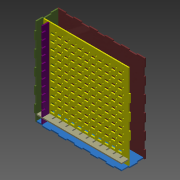
# Autodesk Inventor part: wordClock
Saved by Autodesk Inventor 2015 (Build 190159000, 159)
## iProperties
Created: 2015-02-10
Part Number: wordClock
Material: Generic
Document SubType Name: Modeling
Designer: Iain
Density: 1 g/cm^3
Appearance: Default
Author: Iain
Autodesk Inventor part; units mm, degrees
(part 1 of 2)
ref_plane "YZ Plane" through (0, 0, 0) normal (1, 0, 0) x (0, 1, 0)
ref_plane "XZ Plane" through (0, 0, 0) normal (0, 1, 0) x (-1, 0, 0)
ref_plane "XY Plane" through (0, 0, 0) normal (0, 0, 1) x (1, 0, 0)
sketch "Sketch1" plane through (0, 0, 0) normal (0, 0, 1) x (1, 0, 0)
  line L0 (-105, 105) -> (105, 105)
  line L1 (105, 105) -> (105, -105)
  line L2 (105, -105) -> (-105, -105)
  line L3 (-105, -105) -> (-105, 105)
  point P0 (0, 0)
  point P1 (0, 105)
  point P2 (-105, 0)
  dimension "FrontFaceBaseWidth" = 210
  dimension "FrontFaceBaseHeight" = 210
  constraints: 8 end point, 2 midpoint, 2 parallel, 1 horizontal, 1 horizontal alignment, 1 perpendicular, 1 vertical alignment
  measures "FrontFaceBaseWidth" distance of L0.start L0.end
  measures "FrontFaceBaseHeight" distance of L2.end L0.start
extrude "FrontFaceBase" add sketch "Sketch1" along normal mid plane 3
sketch "Sketch4" plane through (0, 0, 1.5) normal (0, 0, 1) x (1, 0, 0)
  line L0 (-108, 108) -> (-88, 108)
  line L1 (-88, 108) -> (-88, 105)
  line L2 (-88, 105) -> (-108, 105)
  line L3 (-108, 105) -> (-108, 108)
  point P0 (-105, 105)
  point P1 (0, 0)
  point P2 (-98, 105)
  dimension "d6" = 3
  dimension "FrontFaceTabWidth" = 20
  dimension "d8" = 3
  constraints: 8 end point, 2 parallel, 1 horizontal, 1 horizontal alignment, 1 midpoint, 1 perpendicular
  measures "d6" distance of point (-105, 105) L2.end
  measures "FrontFaceTabWidth" distance of L0.end L0.start
  measures "d8" distance of L1.end L0.end
extrude "Extrusion2" add sketch "Sketch4" against normal blind 3
pattern_linear "FrontTopTabs" count 6 spacing 39.2 along (1, 0, 0) of "Extrusion2"
sketch "Sketch5" plane through (0, 0, 1.5) normal (0, 0, 1) x (1, 0, 0)
  line L0 (-108, -108) -> (-105, -108)
  line L1 (-105, -108) -> (-105, -88)
  line L2 (-105, -88) -> (-108, -88)
  line L3 (-108, -88) -> (-108, -108)
  point P0 (-105, -105)
  point P1 (0, 0)
  point P2 (-105, -98)
  dimension "d14" = 3
  dimension "d15" = 3
  dimension "d16" = 20
  constraints: 8 end point, 2 parallel, 1 horizontal, 1 midpoint, 1 perpendicular, 1 vertical alignment
  measures "d14" distance of point (-105, -105) L0.end
  measures "d15" distance of L0.start L0.end
  measures "d16" distance of L2.end L0.start
extrude "Extrusion3" add sketch "Sketch5" against normal blind 3
pattern_linear "FontLeftTabs" count 6 spacing 39.2 along (0, 1, 0) of "Extrusion3"
mirror "FrontBottomTabs" about plane through (0, 0, 0) normal (0, 1, 0) of "Extrusion2", "FrontTopTabs"
mirror "FontRightTabs" about plane through (0, 0, 0) normal (1, 0, 0) of "Extrusion3", "FontLeftTabs"
sketch "Sketch6" plane through (-9.6, 105, -1.5) normal (0, 1, 0) x (1, 0, 0)
  line L0 (-98.4, -3) -> (117.6, -3)
  line L1 (117.6, -3) -> (117.6, 57)
  line L2 (117.6, 57) -> (-98.4, 57)
  line L3 (-98.4, 57) -> (-98.4, -3)
  line L4 (-59.2, -3) -> (-78.4, -3) projected
  line L5 (-98.4, -3) -> (-98.4, 0) projected
  point P0 (-98.4, -3)
  point P1 (117.6, 27)
  point P2 (9.6, -3)
  point P3 (-68.8, -3)
  point P4 (-98.4, 27)
  point P5 (-98.4, -1.5)
  dimension "d68" = 216
  dimension "d69" = 60
  constraints: 8 end point, 5 midpoint, 2 parallel, 1 horizontal, 1 horizontal alignment, 1 perpendicular, 1 vertical alignment
  measures "d68" distance of L0.start L0.end
  measures "d69" distance of L0.end L1.end
extrude "TopFaceBase" add sketch "Sketch6" along normal blind 3 separate body
sketch "Sketch7" plane through (-9.6, 108, -1.5) normal (0, 1, 0) x (1, 0, 0)
  line L0 (-98.4, -3) -> (117.6, -3) projected
  line L1 (-98.4, 57) -> (-98.4, -3) projected
  line L2 (-98.4, -3) -> (-78.4, -3)
  line L3 (-78.4, -3) -> (-78.4, 0)
  line L4 (-78.4, 0) -> (-98.4, 0)
  line L5 (-98.4, 0) -> (-98.4, -3)
  point P0 (9.6, -1.5)
  point P1 (-98.4, 27)
  point P2 (9.6, -3)
  dimension "d25" = 20
  dimension "TopFaceFrontSlotDepth" = 3
  constraints: 8 end point, 2 midpoint, 2 parallel, 1 horizontal, 1 horizontal alignment, 1 perpendicular, 1 vertical alignment
  measures "d25" distance of L3.end L4.end
  measures "TopFaceFrontSlotDepth" distance of L2.start L4.end
extrude "Extrusion5" cut sketch "Sketch7" against normal blind 3 bodies 2
sketch "Sketch8" plane through (-9.6, 108, -1.5) normal (0, 1, 0) x (1, 0, 0)
  line L0 (117.6, -3) -> (114.6, -3)
  line L1 (114.6, -3) -> (114.6, 17)
  line L2 (114.6, 17) -> (117.6, 17)
  line L3 (117.6, 17) -> (117.6, -3)
  point P0 (9.6, -1.5)
  dimension "TopSideSlotWidth" = 20
  dimension "d33" = 3
  constraints: 8 end point, 2 parallel, 1 horizontal, 1 perpendicular
  measures "TopSideSlotWidth" distance of L0.end L1.end
  measures "d33" distance of L0.start L0.end
extrude "Extrusion6" cut sketch "Sketch8" against normal blind 3 bodies 2
pattern_linear "TopFrontSlots" count 6 spacing 39.2 along (1, 0, 0) of "Extrusion5", "Extrusion2" bodies 2
pattern_linear "TopSideRightSlots" count 2 spacing 40 along (0, 0, -1) of "Extrusion6" bodies 2
ref_plane "Work Plane1" through (-48.8, 108, -28.5) normal (0, 0, 1) x (1, 0, 0)
mirror "TopBackSlots" about plane through (-48.8, 108, -28.5) normal (0, 0, 1) of "Extrusion5", "Extrusion2", "TopFrontSlots" bodies 2
ref_plane "Work Plane2" through (0, 105, -18.5) normal (1, 0, 0) x (0, 0, -1)
mirror "TopSideLeftSlots" about plane through (0, 105, -18.5) normal (1, 0, 0) of "Extrusion6", "TopSideRightSlots" bodies 2
sketch "Sketch12" plane through (108, 105, -18.5) normal (1, 0, 0) x (0, 0, -1)
  line L0 (0, 0) -> (20, 0) projected
  line L1 (-20, 0) -> (40, 0)
  line L2 (40, 0) -> (40, -210)
  line L3 (40, -210) -> (-20, -210)
  line L4 (-20, -210) -> (-20, 0)
  line L5 (-17, -95.4) -> (-17, -114.6) projected
  line L6 (-20, -114.6) -> (-20, -95.4) projected
  point P0 (-18.5, -105)
  point P1 (10, 0)
  point P2 (10, 0)
  point P3 (-20, -105)
  point P4 (-17, -105)
  point P5 (-20, -105)
  dimension "SideFaceBaseHeight" = 210
  dimension "SideFaceBaseDepth" = 60
  constraints: 8 end point, 5 midpoint, 2 coincident, 2 parallel, 1 horizontal, 1 perpendicular
  measures "SideFaceBaseHeight" distance of L3.end L1.start
  measures "SideFaceBaseDepth" distance of L1.start L1.end
extrude "RightFaceBase" add sketch "Sketch12" against normal blind 3 separate body
sketch "Sketch13" plane through (108, 105, -18.5) normal (1, 0, 0) x (0, 0, -1)
  line L0 (-20, 0) -> (40, 0) projected
  line L1 (-20, 3) -> (0, 3)
  line L2 (0, 3) -> (0, 0)
  line L3 (0, 0) -> (-20, 0)
  line L4 (-20, 0) -> (-20, 3)
  line L5 (-20, -114.6) -> (-20, -95.4) projected
  point P0 (-18.5, -105)
  point P1 (-10, 0)
  point P2 (10, 0)
  point P3 (-20, 1.5)
  point P4 (-20, -105)
  dimension "SideFaceTabWidth" = 20
  dimension "SideTopTabDepth" = 3
  constraints: 8 end point, 4 midpoint, 2 parallel, 1 horizontal, 1 horizontal alignment, 1 perpendicular, 1 vertical alignment
  measures "SideFaceTabWidth" distance of L1.start L1.end
  measures "SideTopTabDepth" distance of L3.end L1.start
extrude "Extrusion9" add sketch "Sketch13" against normal blind 3 bodies 3
pattern_linear "SideTopTabs" count 2 spacing 40 along (0, 0, -1) of "Extrusion9" bodies 3
mirror "SideBottomTabs" about plane through (0, 0, 0) normal (0, 1, 0) of "Extrusion9", "SideTopTabs" bodies 3
sketch "Sketch14" plane through (108, 105, -18.5) normal (1, 0, 0) x (0, 0, -1)
  line L0 (-20, 3) -> (-20, -213) projected
  line L1 (-20, 3) -> (0, 3) projected
  line L2 (-20, 3) -> (-17, 3)
  line L3 (-17, 3) -> (-17, -17)
  line L4 (-17, -17) -> (-20, -17)
  line L5 (-20, -17) -> (-20, 3)
  point P0 (-18.5, -105)
  point P1 (-18.5, 3)
  point P2 (-10, 3)
  point P3 (-20, -7)
  point P4 (-20, -105)
  dimension "d61" = 3
  dimension "d62" = 20
  constraints: 8 end point, 4 midpoint, 2 parallel, 1 horizontal, 1 horizontal alignment, 1 perpendicular, 1 vertical alignment
  measures "d61" distance of L2.start L2.end
  measures "d62" distance of L4.end L2.start
extrude "Extrusion10" cut sketch "Sketch14" against normal blind 3 bodies 3
pattern_linear "SideFrontSlots" count 6 spacing 39.2 along (0, -1, 0) of "Extrusion10" bodies 3
ref_plane "Work Plane4" through (105, 29.6, -28.5) normal (0, 0, 1) x (1, 0, 0)
mirror "SideBackSlots" about plane through (105, 29.6, -28.5) normal (0, 0, 1) of "Extrusion10", "SideFrontSlots" bodies 3
mirror "Back" about plane through (105, 29.6, -28.5) normal (0, 0, 1) bodies 1 separate body
mirror "Left" about plane through (0, 105, -18.5) normal (1, 0, 0) bodies 3 separate body
mirror "Bottom" about plane through (0, 0, 0) normal (0, 1, 0) bodies 2 separate body
ref_plane "MiddleFacePlane" through (0, 0, -18.5) normal (0, 0, 1) x (1, 0, 0)
sketch "Sketch17" plane through (0, 0, -18.5) normal (0, 0, 1) x (1, 0, 0)
  line L0 (-105, 105) -> (105, 105)
  line L1 (105, 105) -> (105, -105)
  line L2 (105, -105) -> (-105, -105)
  line L3 (-105, -105) -> (-105, 105)
  point P0 (0, 0)
  point P1 (0, 105)
  point P2 (105, 0)
  dimension "d76" = 210
  dimension "d77" = 210
  constraints: 8 end point, 2 midpoint, 2 parallel, 1 horizontal, 1 horizontal alignment, 1 perpendicular, 1 vertical alignment
  measures "d76" distance of L0.end L1.end
  measures "d77" distance of L0.start L0.end
extrude "Extrusion13" add sketch "Sketch17" against normal blind 3 separate body
sketch "Sketch18" plane through (0, 0, -18.5) normal (0, 0, 1) x (1, 0, 0)
  line L0 (-105, -105) -> (-105, 105) projected
  line L1 (-105, -10) -> (-108, -10)
  line L2 (-108, -10) -> (-108, 10)
  line L3 (-108, 10) -> (-105, 10)
  line L4 (-105, 10) -> (-105, -10)
  point P0 (0, 0)
  point P1 (-105, 0)
  point P2 (-105, 0)
  point P3 (-108, 0)
  dimension "d80" = 3
  dimension "MiddleTabWidth" = 20
  constraints: 8 end point, 3 midpoint, 2 parallel, 1 coincident, 1 horizontal, 1 horizontal alignment, 1 perpendicular
  measures "d80" distance of L2.end L3.end
  measures "MiddleTabWidth" distance of L1.end L2.end
extrude "Extrusion14" add sketch "Sketch18" against normal blind 3 bodies 7
pattern_linear "LeftMiddleTabs" count 3 spacing 40 along (0, 1, 0) of "Extrusion14" first direction both ways yes bodies 7
mirror "RightMiddleTabs" about plane through (0, 0, 0) normal (1, 0, 0) of "Extrusion14", "LeftMiddleTabs" bodies 7
sketch "Sketch19" plane through (0, 0, -18.5) normal (0, 0, 1) x (1, 0, 0)
  line L0 (105, -105) -> (-105, -105) projected
  line L1 (-10, -105) -> (10, -105)
  line L2 (10, -105) -> (10, -108)
  line L3 (10, -108) -> (-10, -108)
  line L4 (-10, -108) -> (-10, -105)
  point P0 (0, 0)
  point P1 (0, -105)
  point P2 (0, -105)
  dimension "d87" = 3
  dimension "MiddleBottomTabWidth" = 20
  constraints: 8 end point, 2 midpoint, 2 parallel, 1 coincident, 1 horizontal, 1 perpendicular, 1 vertical alignment
  measures "d87" distance of L1.end L2.end
  measures "MiddleBottomTabWidth" distance of L1.start L1.end
extrude "Extrusion15" add sketch "Sketch19" against normal blind 3 bodies 7
pattern_linear "Rectangular Pattern9" count 3 spacing 40 along (-1, 0, 0) of "Extrusion15" first direction both ways yes bodies 7
sketch "Sketch21" plane through (0, 0, -18.5) normal (0, 0, 1) x (1, 0, 0)
  line L0 (10, -108) -> (-10, -108) projected
  line L1 (-10, -105) -> (10, -105)
  line L2 (10, -105) -> (10, -108)
  line L3 (10, -108) -> (-10, -108)
  line L4 (-10, -108) -> (-10, -105)
  point P0 (0, 0)
  point P1 (0, -105)
  point P2 (0, -108)
  point P3 (0, -108)
  dimension "d94" = 3
  dimension "d95" = 20
  constraints: 8 end point, 3 midpoint, 2 parallel, 1 coincident, 1 horizontal, 1 perpendicular, 1 vertical alignment
  measures "d94" distance of L1.end L2.end
  measures "d95" distance of L1.start L1.end
extrude "Extrusion16" cut sketch "Sketch21" against normal blind 3 bodies 6
pattern_linear "BottomMiddleSlots" count 3 spacing 40 along (-1, 0, 0) of "Extrusion16" first direction both ways yes bodies 6
sketch "Sketch22" plane through (0, 0, -18.5) normal (0, 0, 1) x (1, 0, 0)
  line L0 (-108, -10) -> (-108, 10) projected
  line L1 (-108, 10) -> (-105, 10)
  line L2 (-105, 10) -> (-105, -10)
  line L3 (-105, -10) -> (-108, -10)
  line L4 (-108, -10) -> (-108, 10)
  point P0 (0, 0)
  point P1 (-105, 0)
  point P2 (-108, 0)
  point P3 (-108, 0)
  dimension "d101" = 3
  dimension "d102" = 20
  constraints: 8 end point, 3 midpoint, 2 parallel, 1 coincident, 1 horizontal, 1 horizontal alignment, 1 perpendicular
  measures "d101" distance of L1.end L1.start
  measures "d102" distance of L3.end L1.start
extrude "Extrusion17" cut sketch "Sketch22" against normal blind 3 bodies 5
pattern_linear "LeftMiddleSlots" count 3 spacing 40 along (0, 1, 0) of "Extrusion14", "Extrusion17" first direction both ways yes bodies 5
mirror "RightMiddleSlots" about plane through (0, 0, 0) normal (1, 0, 0) of "LeftMiddleSlots", "Extrusion14", "Extrusion17" bodies 3
sketch "gridConstruct" plane through (0, 0, 1.5) normal (0, 0, 1) x (1, 0, 0)
  line L0 (88, 108) -> (108, 108) projected
  line L1 (88, 105) -> (88, 108) projected
  line L2 (88, 105) -> (68.8, 105) projected
  line L3 (68.8, 108) -> (68.8, 105) projected
  line L4 (48.8, 108) -> (68.8, 108) projected
  line L5 (48.8, 105) -> (48.8, 108) projected
  line L6 (48.8, 105) -> (29.6, 105) projected
  line L7 (29.6, 108) -> (29.6, 105) projected
  line L8 (9.6, 108) -> (29.6, 108) projected
  line L9 (9.6, 105) -> (9.6, 108) projected
  line L10 (9.6, 105) -> (-9.6, 105) projected
  line L11 (-9.6, 108) -> (-9.6, 105) projected
  line L12 (-29.6, 108) -> (-9.6, 108) projected
  line L13 (-29.6, 105) -> (-29.6, 108) projected
  line L14 (-29.6, 105) -> (-48.8, 105) projected
  line L15 (-48.8, 108) -> (-48.8, 105) projected
  line L16 (-68.8, 108) -> (-48.8, 108) projected
  line L17 (-68.8, 105) -> (-68.8, 108) projected
  line L18 (-68.8, 105) -> (-88, 105) projected
  line L19 (-88, 108) -> (-88, 105) projected
  line L20 (-108, 108) -> (-88, 108) projected
  line L21 (-108, 108) -> (-108, 88) projected
  line L22 (-108, 88) -> (-105, 88) projected
  line L23 (-105, 88) -> (-105, 68.8) projected
  line L24 (-105, 68.8) -> (-108, 68.8) projected
  line L25 (-108, 68.8) -> (-108, 48.8) projected
  line L26 (-108, 48.8) -> (-105, 48.8) projected
  line L27 (-105, 48.8) -> (-105, 29.6) projected
  line L28 (-105, 29.6) -> (-108, 29.6) projected
  line L29 (-108, 29.6) -> (-108, 9.6) projected
  line L30 (-108, 9.6) -> (-105, 9.6) projected
  line L31 (-105, 9.6) -> (-105, -9.6) projected
  line L32 (-105, -9.6) -> (-108, -9.6) projected
  line L33 (-108, -9.6) -> (-108, -29.6) projected
  line L34 (-108, -29.6) -> (-105, -29.6) projected
  line L35 (-105, -29.6) -> (-105, -48.8) projected
  line L36 (-105, -48.8) -> (-108, -48.8) projected
  line L37 (-108, -48.8) -> (-108, -68.8) projected
  line L38 (-108, -68.8) -> (-105, -68.8) projected
  line L39 (-105, -68.8) -> (-105, -88) projected
  line L40 (-105, -88) -> (-108, -88) projected
  line L41 (-108, -88) -> (-108, -108) projected
  line L42 (-108, -108) -> (-88, -108) projected
  line L43 (-88, -108) -> (-88, -105) projected
  line L44 (-88, -105) -> (-68.8, -105) projected
  line L45 (-68.8, -105) -> (-68.8, -108) projected
  line L46 (-68.8, -108) -> (-48.8, -108) projected
  line L47 (-48.8, -108) -> (-48.8, -105) projected
  line L48 (-48.8, -105) -> (-29.6, -105) projected
  line L49 (-29.6, -105) -> (-29.6, -108) projected
  line L50 (-29.6, -108) -> (-9.6, -108) projected
  line L51 (-9.6, -108) -> (-9.6, -105) projected
  line L52 (-9.6, -105) -> (9.6, -105) projected
  line L53 (9.6, -105) -> (9.6, -108) projected
  line L54 (9.6, -108) -> (29.6, -108) projected
  line L55 (29.6, -108) -> (29.6, -105) projected
  line L56 (29.6, -105) -> (48.8, -105) projected
  line L57 (48.8, -105) -> (48.8, -108) projected
  line L58 (48.8, -108) -> (68.8, -108) projected
  line L59 (68.8, -108) -> (68.8, -105) projected
  line L60 (68.8, -105) -> (88, -105) projected
  line L61 (88, -105) -> (88, -108) projected
  line L62 (88, -108) -> (108, -108) projected
  line L63 (108, -108) -> (108, -88) projected
  line L64 (105, -88) -> (108, -88) projected
  line L65 (105, -88) -> (105, -68.8) projected
  line L66 (108, -68.8) -> (105, -68.8) projected
  line L67 (108, -48.8) -> (108, -68.8) projected
  line L68 (105, -48.8) -> (108, -48.8) projected
  line L69 (105, -48.8) -> (105, -29.6) projected
  line L70 (108, -29.6) -> (105, -29.6) projected
  line L71 (108, -9.6) -> (108, -29.6) projected
  line L72 (105, -9.6) -> (108, -9.6) projected
  line L73 (105, -9.6) -> (105, 9.6) projected
  line L74 (108, 9.6) -> (105, 9.6) projected
  line L75 (108, 29.6) -> (108, 9.6) projected
  line L76 (105, 29.6) -> (108, 29.6) projected
  line L77 (105, 29.6) -> (105, 48.8) projected
  line L78 (108, 48.8) -> (105, 48.8) projected
  line L79 (108, 68.8) -> (108, 48.8) projected
  line L80 (105, 68.8) -> (108, 68.8) projected
  line L81 (105, 68.8) -> (105, 88) projected
  line L82 (108, 88) -> (105, 88) projected
  line L83 (108, 108) -> (108, 88) projected
  line L84 (-91.6667, -75) -> (-75, -75) construction
  line L85 (-75, -75) -> (-75, -91.6667) construction
  line L86 (-75, -91.6667) -> (-91.6667, -91.6667) construction
  line L87 (-91.6667, -91.6667) -> (-91.6667, -75) construction
  line L88 (-75, -75) -> (-58.3333, -75) construction
  line L89 (-58.3333, -75) -> (-58.3333, -91.6667) construction
  line L90 (-58.3333, -91.6667) -> (-75, -91.6667) construction
  line L91 (-75, -91.6667) -> (-75, -75) construction
  line L92 (-58.3333, -75) -> (-41.6667, -75) construction
  line L93 (-41.6667, -75) -> (-41.6667, -91.6667) construction
  line L94 (-41.6667, -91.6667) -> (-58.3333, -91.6667) construction
  line L95 (-58.3333, -91.6667) -> (-58.3333, -75) construction
  line L96 (-41.6667, -75) -> (-25, -75) construction
  line L97 (-25, -75) -> (-25, -91.6667) construction
  line L98 (-25, -91.6667) -> (-41.6667, -91.6667) construction
  line L99 (-41.6667, -91.6667) -> (-41.6667, -75) construction
  line L100 (-25, -75) -> (-8.3333, -75) construction
  line L101 (-8.3333, -75) -> (-8.3333, -91.6667) construction
  line L102 (-8.3333, -91.6667) -> (-25, -91.6667) construction
  line L103 (-25, -91.6667) -> (-25, -75) construction
  line L104 (-8.3333, -75) -> (8.3333, -75) construction
  line L105 (8.3333, -75) -> (8.3333, -91.6667) construction
  line L106 (8.3333, -91.6667) -> (-8.3333, -91.6667) construction
  line L107 (-8.3333, -91.6667) -> (-8.3333, -75) construction
  line L108 (-91.6667, -58.3333) -> (-75, -58.3333) construction
  line L109 (-75, -58.3333) -> (-75, -75) construction
  line L110 (-75, -75) -> (-91.6667, -75) construction
  line L111 (-91.6667, -75) -> (-91.6667, -58.3333) construction
  line L112 (-75, -58.3333) -> (-58.3333, -58.3333) construction
  line L113 (-58.3333, -58.3333) -> (-58.3333, -75) construction
  line L114 (-58.3333, -75) -> (-75, -75) construction
  line L115 (-75, -75) -> (-75, -58.3333) construction
  line L116 (-58.3333, -58.3333) -> (-41.6667, -58.3333) construction
  line L117 (-41.6667, -58.3333) -> (-41.6667, -75) construction
  line L118 (-41.6667, -75) -> (-58.3333, -75) construction
  line L119 (-58.3333, -75) -> (-58.3333, -58.3333) construction
  line L120 (-41.6667, -58.3333) -> (-25, -58.3333) construction
  line L121 (-25, -58.3333) -> (-25, -75) construction
  line L122 (-25, -75) -> (-41.6667, -75) construction
  line L123 (-41.6667, -75) -> (-41.6667, -58.3333) construction
  line L124 (-25, -58.3333) -> (-8.3333, -58.3333) construction
  line L125 (-8.3333, -58.3333) -> (-8.3333, -75) construction
  line L126 (-8.3333, -75) -> (-25, -75) construction
  line L127 (-25, -75) -> (-25, -58.3333) construction
  line L128 (-8.3333, -58.3333) -> (8.3333, -58.3333) construction
  line L129 (8.3333, -58.3333) -> (8.3333, -75) construction
  line L130 (8.3333, -75) -> (-8.3333, -75) construction
  line L131 (-8.3333, -75) -> (-8.3333, -58.3333) construction
  line L132 (-91.6667, -41.6667) -> (-75, -41.6667) construction
  line L133 (-75, -41.6667) -> (-75, -58.3333) construction
  line L134 (-75, -58.3333) -> (-91.6667, -58.3333) construction
  line L135 (-91.6667, -58.3333) -> (-91.6667, -41.6667) construction
  line L136 (-75, -41.6667) -> (-58.3333, -41.6667) construction
  line L137 (-58.3333, -41.6667) -> (-58.3333, -58.3333) construction
  line L138 (-58.3333, -58.3333) -> (-75, -58.3333) construction
  line L139 (-75, -58.3333) -> (-75, -41.6667) construction
  line L140 (-58.3333, -41.6667) -> (-41.6667, -41.6667) construction
  line L141 (-41.6667, -41.6667) -> (-41.6667, -58.3333) construction
  line L142 (-41.6667, -58.3333) -> (-58.3333, -58.3333) construction
  line L143 (-58.3333, -58.3333) -> (-58.3333, -41.6667) construction
  line L144 (-41.6667, -41.6667) -> (-25, -41.6667) construction
  line L145 (-25, -41.6667) -> (-25, -58.3333) construction
  line L146 (-25, -58.3333) -> (-41.6667, -58.3333) construction
  line L147 (-41.6667, -58.3333) -> (-41.6667, -41.6667) construction
  line L148 (-25, -41.6667) -> (-8.3333, -41.6667) construction
  line L149 (-8.3333, -41.6667) -> (-8.3333, -58.3333) construction
  line L150 (-8.3333, -58.3333) -> (-25, -58.3333) construction
  line L151 (-25, -58.3333) -> (-25, -41.6667) construction
  line L152 (-8.3333, -41.6667) -> (8.3333, -41.6667) construction
  line L153 (8.3333, -41.6667) -> (8.3333, -58.3333) construction
  line L154 (8.3333, -58.3333) -> (-8.3333, -58.3333) construction
  line L155 (-8.3333, -58.3333) -> (-8.3333, -41.6667) construction
  line L156 (-91.6667, -25) -> (-75, -25) construction
  line L157 (-75, -25) -> (-75, -41.6667) construction
  line L158 (-75, -41.6667) -> (-91.6667, -41.6667) construction
  line L159 (-91.6667, -41.6667) -> (-91.6667, -25) construction
  line L160 (-75, -25) -> (-58.3333, -25) construction
  line L161 (-58.3333, -25) -> (-58.3333, -41.6667) construction
  line L162 (-58.3333, -41.6667) -> (-75, -41.6667) construction
  line L163 (-75, -41.6667) -> (-75, -25) construction
  line L164 (-58.3333, -25) -> (-41.6667, -25) construction
  line L165 (-41.6667, -25) -> (-41.6667, -41.6667) construction
  line L166 (-41.6667, -41.6667) -> (-58.3333, -41.6667) construction
  line L167 (-58.3333, -41.6667) -> (-58.3333, -25) construction
  line L168 (-41.6667, -25) -> (-25, -25) construction
  line L169 (-25, -25) -> (-25, -41.6667) construction
  line L170 (-25, -41.6667) -> (-41.6667, -41.6667) construction
  line L171 (-41.6667, -41.6667) -> (-41.6667, -25) construction
  line L172 (-25, -25) -> (-8.3333, -25) construction
  line L173 (-8.3333, -25) -> (-8.3333, -41.6667) construction
  line L174 (-8.3333, -41.6667) -> (-25, -41.6667) construction
  line L175 (-25, -41.6667) -> (-25, -25) construction
  line L176 (-8.3333, -25) -> (8.3333, -25) construction
  line L177 (8.3333, -25) -> (8.3333, -41.6667) construction
  line L178 (8.3333, -41.6667) -> (-8.3333, -41.6667) construction
  line L179 (-8.3333, -41.6667) -> (-8.3333, -25) construction
  line L180 (-91.6667, -8.3333) -> (-75, -8.3333) construction
  line L181 (-75, -8.3333) -> (-75, -25) construction
  line L182 (-75, -25) -> (-91.6667, -25) construction
  line L183 (-91.6667, -25) -> (-91.6667, -8.3333) construction
  line L184 (-75, -8.3333) -> (-58.3333, -8.3333) construction
  line L185 (-58.3333, -8.3333) -> (-58.3333, -25) construction
  line L186 (-58.3333, -25) -> (-75, -25) construction
  line L187 (-75, -25) -> (-75, -8.3333) construction
  line L188 (-58.3333, -8.3333) -> (-41.6667, -8.3333) construction
  line L189 (-41.6667, -8.3333) -> (-41.6667, -25) construction
  line L190 (-41.6667, -25) -> (-58.3333, -25) construction
  line L191 (-58.3333, -25) -> (-58.3333, -8.3333) construction
  line L192 (-41.6667, -8.3333) -> (-25, -8.3333) construction
  line L193 (-25, -8.3333) -> (-25, -25) construction
  line L194 (-25, -25) -> (-41.6667, -25) construction
  line L195 (-41.6667, -25) -> (-41.6667, -8.3333) construction
  line L196 (-25, -8.3333) -> (-8.3333, -8.3333) construction
  line L197 (-8.3333, -8.3333) -> (-8.3333, -25) construction
  line L198 (-8.3333, -25) -> (-25, -25) construction
  line L199 (-25, -25) -> (-25, -8.3333) construction
  line L200 (-8.3333, -8.3333) -> (8.3333, -8.3333) construction
  line L201 (8.3333, -8.3333) -> (8.3333, -25) construction
  line L202 (8.3333, -25) -> (-8.3333, -25) construction
  line L203 (-8.3333, -25) -> (-8.3333, -8.3333) construction
  line L204 (-91.6667, 8.3333) -> (-75, 8.3333) construction
  line L205 (-75, 8.3333) -> (-75, -8.3333) construction
  line L206 (-75, -8.3333) -> (-91.6667, -8.3333) construction
  line L207 (-91.6667, -8.3333) -> (-91.6667, 8.3333) construction
  line L208 (-75, 8.3333) -> (-58.3333, 8.3333) construction
  line L209 (-58.3333, 8.3333) -> (-58.3333, -8.3333) construction
  line L210 (-58.3333, -8.3333) -> (-75, -8.3333) construction
  line L211 (-75, -8.3333) -> (-75, 8.3333) construction
  line L212 (-58.3333, 8.3333) -> (-41.6667, 8.3333) construction
  line L213 (-41.6667, 8.3333) -> (-41.6667, -8.3333) construction
  line L214 (-41.6667, -8.3333) -> (-58.3333, -8.3333) construction
  line L215 (-58.3333, -8.3333) -> (-58.3333, 8.3333) construction
  line L216 (-41.6667, 8.3333) -> (-25, 8.3333) construction
  line L217 (-25, 8.3333) -> (-25, -8.3333) construction
  line L218 (-25, -8.3333) -> (-41.6667, -8.3333) construction
  line L219 (-41.6667, -8.3333) -> (-41.6667, 8.3333) construction
  line L220 (-25, 8.3333) -> (-8.3333, 8.3333) construction
  line L221 (-8.3333, 8.3333) -> (-8.3333, -8.3333) construction
  line L222 (-8.3333, -8.3333) -> (-25, -8.3333) construction
  line L223 (-25, -8.3333) -> (-25, 8.3333) construction
  line L224 (-8.3333, 8.3333) -> (8.3333, 8.3333) construction
  line L225 (8.3333, 8.3333) -> (8.3333, -8.3333) construction
  line L226 (8.3333, -8.3333) -> (-8.3333, -8.3333) construction
  line L227 (-8.3333, -8.3333) -> (-8.3333, 8.3333) construction
  line L228 (-91.6667, 25) -> (-75, 25) construction
  line L229 (-75, 25) -> (-75, 8.3333) construction
  line L230 (-75, 8.3333) -> (-91.6667, 8.3333) construction
  line L231 (-91.6667, 8.3333) -> (-91.6667, 25) construction
  line L232 (-75, 25) -> (-58.3333, 25) construction
  line L233 (-58.3333, 25) -> (-58.3333, 8.3333) construction
  line L234 (-58.3333, 8.3333) -> (-75, 8.3333) construction
  line L235 (-75, 8.3333) -> (-75, 25) construction
  line L236 (-58.3333, 25) -> (-41.6667, 25) construction
  line L237 (-41.6667, 25) -> (-41.6667, 8.3333) construction
  line L238 (-41.6667, 8.3333) -> (-58.3333, 8.3333) construction
  line L239 (-58.3333, 8.3333) -> (-58.3333, 25) construction
  line L240 (-41.6667, 25) -> (-25, 25) construction
  line L241 (-25, 25) -> (-25, 8.3333) construction
  line L242 (-25, 8.3333) -> (-41.6667, 8.3333) construction
  line L243 (-41.6667, 8.3333) -> (-41.6667, 25) construction
  line L244 (-25, 25) -> (-8.3333, 25) construction
  line L245 (-8.3333, 25) -> (-8.3333, 8.3333) construction
  line L246 (-8.3333, 8.3333) -> (-25, 8.3333) construction
  line L247 (-25, 8.3333) -> (-25, 25) construction
  line L248 (-8.3333, 25) -> (8.3333, 25) construction
  line L249 (8.3333, 25) -> (8.3333, 8.3333) construction
  line L250 (8.3333, 8.3333) -> (-8.3333, 8.3333) construction
  line L251 (-8.3333, 8.3333) -> (-8.3333, 25) construction
  line L252 (-91.6667, 41.6667) -> (-75, 41.6667) construction
  line L253 (-75, 41.6667) -> (-75, 25) construction
  line L254 (-75, 25) -> (-91.6667, 25) construction
  line L255 (-91.6667, 25) -> (-91.6667, 41.6667) construction
  line L256 (-75, 41.6667) -> (-58.3333, 41.6667) construction
  line L257 (-58.3333, 41.6667) -> (-58.3333, 25) construction
  line L258 (-58.3333, 25) -> (-75, 25) construction
  line L259 (-75, 25) -> (-75, 41.6667) construction
  line L260 (-58.3333, 41.6667) -> (-41.6667, 41.6667) construction
  line L261 (-41.6667, 41.6667) -> (-41.6667, 25) construction
  line L262 (-41.6667, 25) -> (-58.3333, 25) construction
  line L263 (-58.3333, 25) -> (-58.3333, 41.6667) construction
  line L264 (-41.6667, 41.6667) -> (-25, 41.6667) construction
  line L265 (-25, 41.6667) -> (-25, 25) construction
  line L266 (-25, 25) -> (-41.6667, 25) construction
  line L267 (-41.6667, 25) -> (-41.6667, 41.6667) construction
  line L268 (-25, 41.6667) -> (-8.3333, 41.6667) construction
  line L269 (-8.3333, 41.6667) -> (-8.3333, 25) construction
  line L270 (-8.3333, 25) -> (-25, 25) construction
  line L271 (-25, 25) -> (-25, 41.6667) construction
  line L272 (-8.3333, 41.6667) -> (8.3333, 41.6667) construction
  line L273 (8.3333, 41.6667) -> (8.3333, 25) construction
  line L274 (8.3333, 25) -> (-8.3333, 25) construction
  line L275 (-8.3333, 25) -> (-8.3333, 41.6667) construction
  line L276 (-91.6667, 58.3333) -> (-75, 58.3333) construction
  line L277 (-75, 58.3333) -> (-75, 41.6667) construction
  line L278 (-75, 41.6667) -> (-91.6667, 41.6667) construction
  line L279 (-91.6667, 41.6667) -> (-91.6667, 58.3333) construction
  line L280 (-75, 58.3333) -> (-58.3333, 58.3333) construction
  line L281 (-58.3333, 58.3333) -> (-58.3333, 41.6667) construction
  line L282 (-58.3333, 41.6667) -> (-75, 41.6667) construction
  line L283 (-75, 41.6667) -> (-75, 58.3333) construction
  line L284 (-58.3333, 58.3333) -> (-41.6667, 58.3333) construction
  line L285 (-41.6667, 58.3333) -> (-41.6667, 41.6667) construction
  line L286 (-41.6667, 41.6667) -> (-58.3333, 41.6667) construction
  line L287 (-58.3333, 41.6667) -> (-58.3333, 58.3333) construction
  line L288 (-41.6667, 58.3333) -> (-25, 58.3333) construction
  line L289 (-25, 58.3333) -> (-25, 41.6667) construction
  line L290 (-25, 41.6667) -> (-41.6667, 41.6667) construction
  line L291 (-41.6667, 41.6667) -> (-41.6667, 58.3333) construction
  line L292 (-25, 58.3333) -> (-8.3333, 58.3333) construction
  line L293 (-8.3333, 58.3333) -> (-8.3333, 41.6667) construction
  line L294 (-8.3333, 41.6667) -> (-25, 41.6667) construction
  line L295 (-25, 41.6667) -> (-25, 58.3333) construction
  line L296 (-8.3333, 58.3333) -> (8.3333, 58.3333) construction
  line L297 (8.3333, 58.3333) -> (8.3333, 41.6667) construction
  line L298 (8.3333, 41.6667) -> (-8.3333, 41.6667) construction
  line L299 (-8.3333, 41.6667) -> (-8.3333, 58.3333) construction
  line L300 (8.3333, -75) -> (25, -75) construction
  line L301 (25, -75) -> (25, -91.6667) construction
  line L302 (25, -91.6667) -> (8.3333, -91.6667) construction
  line L303 (8.3333, -91.6667) -> (8.3333, -75) construction
  line L304 (8.3333, -58.3333) -> (25, -58.3333) construction
  line L305 (25, -58.3333) -> (25, -75) construction
  line L306 (25, -75) -> (8.3333, -75) construction
  line L307 (8.3333, -75) -> (8.3333, -58.3333) construction
  line L308 (8.3333, -41.6667) -> (25, -41.6667) construction
  line L309 (25, -41.6667) -> (25, -58.3333) construction
  line L310 (25, -58.3333) -> (8.3333, -58.3333) construction
  line L311 (8.3333, -58.3333) -> (8.3333, -41.6667) construction
  line L312 (8.3333, -25) -> (25, -25) construction
  line L313 (25, -25) -> (25, -41.6667) construction
  line L314 (25, -41.6667) -> (8.3333, -41.6667) construction
  line L315 (8.3333, -41.6667) -> (8.3333, -25) construction
  line L316 (8.3333, -8.3333) -> (25, -8.3333) construction
  line L317 (25, -8.3333) -> (25, -25) construction
  line L318 (25, -25) -> (8.3333, -25) construction
  line L319 (8.3333, -25) -> (8.3333, -8.3333) construction
  line L320 (8.3333, 8.3333) -> (25, 8.3333) construction
  line L321 (25, 8.3333) -> (25, -8.3333) construction
  line L322 (25, -8.3333) -> (8.3333, -8.3333) construction
  line L323 (8.3333, -8.3333) -> (8.3333, 8.3333) construction
  line L324 (8.3333, 25) -> (25, 25) construction
  line L325 (25, 25) -> (25, 8.3333) construction
  line L326 (25, 8.3333) -> (8.3333, 8.3333) construction
  line L327 (8.3333, 8.3333) -> (8.3333, 25) construction
  line L328 (8.3333, 41.6667) -> (25, 41.6667) construction
  line L329 (25, 41.6667) -> (25, 25) construction
  line L330 (25, 25) -> (8.3333, 25) construction
  line L331 (8.3333, 25) -> (8.3333, 41.6667) construction
  line L332 (8.3333, 58.3333) -> (25, 58.3333) construction
  line L333 (25, 58.3333) -> (25, 41.6667) construction
  line L334 (25, 41.6667) -> (8.3333, 41.6667) construction
  line L335 (8.3333, 41.6667) -> (8.3333, 58.3333) construction
  line L336 (25, -75) -> (41.6667, -75) construction
  line L337 (41.6667, -75) -> (41.6667, -91.6667) construction
  line L338 (41.6667, -91.6667) -> (25, -91.6667) construction
  line L339 (25, -91.6667) -> (25, -75) construction
  line L340 (25, -58.3333) -> (41.6667, -58.3333) construction
  line L341 (41.6667, -58.3333) -> (41.6667, -75) construction
  line L342 (41.6667, -75) -> (25, -75) construction
  line L343 (25, -75) -> (25, -58.3333) construction
  line L344 (25, -41.6667) -> (41.6667, -41.6667) construction
  line L345 (41.6667, -41.6667) -> (41.6667, -58.3333) construction
  line L346 (41.6667, -58.3333) -> (25, -58.3333) construction
  line L347 (25, -58.3333) -> (25, -41.6667) construction
  line L348 (25, -25) -> (41.6667, -25) construction
  line L349 (41.6667, -25) -> (41.6667, -41.6667) construction
  line L350 (41.6667, -41.6667) -> (25, -41.6667) construction
  line L351 (25, -41.6667) -> (25, -25) construction
  line L352 (25, -8.3333) -> (41.6667, -8.3333) construction
  line L353 (41.6667, -8.3333) -> (41.6667, -25) construction
  line L354 (41.6667, -25) -> (25, -25) construction
  line L355 (25, -25) -> (25, -8.3333) construction
  line L356 (25, 8.3333) -> (41.6667, 8.3333) construction
  line L357 (41.6667, 8.3333) -> (41.6667, -8.3333) construction
  line L358 (41.6667, -8.3333) -> (25, -8.3333) construction
  line L359 (25, -8.3333) -> (25, 8.3333) construction
  line L360 (25, 25) -> (41.6667, 25) construction
  line L361 (41.6667, 25) -> (41.6667, 8.3333) construction
  line L362 (41.6667, 8.3333) -> (25, 8.3333) construction
  line L363 (25, 8.3333) -> (25, 25) construction
  line L364 (25, 41.6667) -> (41.6667, 41.6667) construction
  line L365 (41.6667, 41.6667) -> (41.6667, 25) construction
  line L366 (41.6667, 25) -> (25, 25) construction
  line L367 (25, 25) -> (25, 41.6667) construction
  line L368 (25, 58.3333) -> (41.6667, 58.3333) construction
  line L369 (41.6667, 58.3333) -> (41.6667, 41.6667) construction
  line L370 (41.6667, 41.6667) -> (25, 41.6667) construction
  line L371 (25, 41.6667) -> (25, 58.3333) construction
  line L372 (41.6667, -75) -> (58.3333, -75) construction
  line L373 (58.3333, -75) -> (58.3333, -91.6667) construction
  line L374 (58.3333, -91.6667) -> (41.6667, -91.6667) construction
  line L375 (41.6667, -91.6667) -> (41.6667, -75) construction
  line L376 (41.6667, -58.3333) -> (58.3333, -58.3333) construction
  line L377 (58.3333, -58.3333) -> (58.3333, -75) construction
  line L378 (58.3333, -75) -> (41.6667, -75) construction
  line L379 (41.6667, -75) -> (41.6667, -58.3333) construction
  line L380 (41.6667, -41.6667) -> (58.3333, -41.6667) construction
  line L381 (58.3333, -41.6667) -> (58.3333, -58.3333) construction
  line L382 (58.3333, -58.3333) -> (41.6667, -58.3333) construction
  line L383 (41.6667, -58.3333) -> (41.6667, -41.6667) construction
  line L384 (41.6667, -25) -> (58.3333, -25) construction
  line L385 (58.3333, -25) -> (58.3333, -41.6667) construction
  line L386 (58.3333, -41.6667) -> (41.6667, -41.6667) construction
  line L387 (41.6667, -41.6667) -> (41.6667, -25) construction
  line L388 (41.6667, -8.3333) -> (58.3333, -8.3333) construction
  line L389 (58.3333, -8.3333) -> (58.3333, -25) construction
  line L390 (58.3333, -25) -> (41.6667, -25) construction
  line L391 (41.6667, -25) -> (41.6667, -8.3333) construction
  line L392 (41.6667, 8.3333) -> (58.3333, 8.3333) construction
  line L393 (58.3333, 8.3333) -> (58.3333, -8.3333) construction
  line L394 (58.3333, -8.3333) -> (41.6667, -8.3333) construction
  line L395 (41.6667, -8.3333) -> (41.6667, 8.3333) construction
  line L396 (41.6667, 25) -> (58.3333, 25) construction
  line L397 (58.3333, 25) -> (58.3333, 8.3333) construction
  line L398 (58.3333, 8.3333) -> (41.6667, 8.3333) construction
  line L399 (41.6667, 8.3333) -> (41.6667, 25) construction
  line L400 (41.6667, 41.6667) -> (58.3333, 41.6667) construction
  line L401 (58.3333, 41.6667) -> (58.3333, 25) construction
  line L402 (58.3333, 25) -> (41.6667, 25) construction
  line L403 (41.6667, 25) -> (41.6667, 41.6667) construction
  line L404 (41.6667, 58.3333) -> (58.3333, 58.3333) construction
  line L405 (58.3333, 58.3333) -> (58.3333, 41.6667) construction
  line L406 (58.3333, 41.6667) -> (41.6667, 41.6667) construction
  line L407 (41.6667, 41.6667) -> (41.6667, 58.3333) construction
  line L408 (58.3333, -75) -> (75, -75) construction
  line L409 (75, -75) -> (75, -91.6667) construction
  line L410 (75, -91.6667) -> (58.3333, -91.6667) construction
  line L411 (58.3333, -91.6667) -> (58.3333, -75) construction
  line L412 (58.3333, -58.3333) -> (75, -58.3333) construction
  line L413 (75, -58.3333) -> (75, -75) construction
  line L414 (75, -75) -> (58.3333, -75) construction
  line L415 (58.3333, -75) -> (58.3333, -58.3333) construction
  line L416 (58.3333, -41.6667) -> (75, -41.6667) construction
  line L417 (75, -41.6667) -> (75, -58.3333) construction
  line L418 (75, -58.3333) -> (58.3333, -58.3333) construction
  line L419 (58.3333, -58.3333) -> (58.3333, -41.6667) construction
  line L420 (58.3333, -25) -> (75, -25) construction
  line L421 (75, -25) -> (75, -41.6667) construction
  line L422 (75, -41.6667) -> (58.3333, -41.6667) construction
  line L423 (58.3333, -41.6667) -> (58.3333, -25) construction
  line L424 (58.3333, -8.3333) -> (75, -8.3333) construction
  line L425 (75, -8.3333) -> (75, -25) construction
  line L426 (75, -25) -> (58.3333, -25) construction
  line L427 (58.3333, -25) -> (58.3333, -8.3333) construction
  line L428 (58.3333, 8.3333) -> (75, 8.3333) construction
  line L429 (75, 8.3333) -> (75, -8.3333) construction
  line L430 (75, -8.3333) -> (58.3333, -8.3333) construction
  line L431 (58.3333, -8.3333) -> (58.3333, 8.3333) construction
  line L432 (58.3333, 25) -> (75, 25) construction
  line L433 (75, 25) -> (75, 8.3333) construction
  line L434 (75, 8.3333) -> (58.3333, 8.3333) construction
  line L435 (58.3333, 8.3333) -> (58.3333, 25) construction
  line L436 (58.3333, 41.6667) -> (75, 41.6667) construction
  line L437 (75, 41.6667) -> (75, 25) construction
  line L438 (75, 25) -> (58.3333, 25) construction
  line L439 (58.3333, 25) -> (58.3333, 41.6667) construction
  line L440 (58.3333, 58.3333) -> (75, 58.3333) construction
  line L441 (75, 58.3333) -> (75, 41.6667) construction
  line L442 (75, 41.6667) -> (58.3333, 41.6667) construction
  line L443 (58.3333, 41.6667) -> (58.3333, 58.3333) construction
  line L444 (75, -75) -> (91.6667, -75) construction
  line L445 (91.6667, -75) -> (91.6667, -91.6667) construction
  line L446 (91.6667, -91.6667) -> (75, -91.6667) construction
  line L447 (75, -91.6667) -> (75, -75) construction
  line L448 (75, -58.3333) -> (91.6667, -58.3333) construction
  line L449 (91.6667, -58.3333) -> (91.6667, -75) construction
  line L450 (91.6667, -75) -> (75, -75) construction
  line L451 (75, -75) -> (75, -58.3333) construction
  line L452 (75, -41.6667) -> (91.6667, -41.6667) construction
  line L453 (91.6667, -41.6667) -> (91.6667, -58.3333) construction
  line L454 (91.6667, -58.3333) -> (75, -58.3333) construction
  line L455 (75, -58.3333) -> (75, -41.6667) construction
  line L456 (75, -25) -> (91.6667, -25) construction
  line L457 (91.6667, -25) -> (91.6667, -41.6667) construction
  line L458 (91.6667, -41.6667) -> (75, -41.6667) construction
  line L459 (75, -41.6667) -> (75, -25) construction
  line L460 (75, -8.3333) -> (91.6667, -8.3333) construction
  line L461 (91.6667, -8.3333) -> (91.6667, -25) construction
  line L462 (91.6667, -25) -> (75, -25) construction
  line L463 (75, -25) -> (75, -8.3333) construction
  line L464 (75, 8.3333) -> (91.6667, 8.3333) construction
  line L465 (91.6667, 8.3333) -> (91.6667, -8.3333) construction
  line L466 (91.6667, -8.3333) -> (75, -8.3333) construction
  line L467 (75, -8.3333) -> (75, 8.3333) construction
  line L468 (75, 25) -> (91.6667, 25) construction
  line L469 (91.6667, 25) -> (91.6667, 8.3333) construction
  line L470 (91.6667, 8.3333) -> (75, 8.3333) construction
  line L471 (75, 8.3333) -> (75, 25) construction
  line L472 (75, 41.6667) -> (91.6667, 41.6667) construction
  line L473 (91.6667, 41.6667) -> (91.6667, 25) construction
  line L474 (91.6667, 25) -> (75, 25) construction
  line L475 (75, 25) -> (75, 41.6667) construction
  line L476 (75, 58.3333) -> (91.6667, 58.3333) construction
  line L477 (91.6667, 58.3333) -> (91.6667, 41.6667) construction
  line L478 (91.6667, 41.6667) -> (75, 41.6667) construction
  line L479 (75, 41.6667) -> (75, 58.3333) construction
  line L480 (-91.6667, 75) -> (-75, 75) construction
  line L481 (-75, 75) -> (-75, 58.3333) construction
  line L482 (-75, 58.3333) -> (-91.6667, 58.3333) construction
  line L483 (-91.6667, 58.3333) -> (-91.6667, 75) construction
  line L484 (-75, 75) -> (-58.3333, 75) construction
  line L485 (-58.3333, 75) -> (-58.3333, 58.3333) construction
  line L486 (-58.3333, 58.3333) -> (-75, 58.3333) construction
  line L487 (-75, 58.3333) -> (-75, 75) construction
  line L488 (-58.3333, 75) -> (-41.6667, 75) construction
  line L489 (-41.6667, 75) -> (-41.6667, 58.3333) construction
  line L490 (-41.6667, 58.3333) -> (-58.3333, 58.3333) construction
  line L491 (-58.3333, 58.3333) -> (-58.3333, 75) construction
  line L492 (-41.6667, 75) -> (-25, 75) construction
  line L493 (-25, 75) -> (-25, 58.3333) construction
  line L494 (-25, 58.3333) -> (-41.6667, 58.3333) construction
  line L495 (-41.6667, 58.3333) -> (-41.6667, 75) construction
  line L496 (-25, 75) -> (-8.3333, 75) construction
  line L497 (-8.3333, 75) -> (-8.3333, 58.3333) construction
  line L498 (-8.3333, 58.3333) -> (-25, 58.3333) construction
  line L499 (-25, 58.3333) -> (-25, 75) construction
  line L500 (-8.3333, 75) -> (8.3333, 75) construction
  line L501 (8.3333, 75) -> (8.3333, 58.3333) construction
  line L502 (8.3333, 58.3333) -> (-8.3333, 58.3333) construction
  line L503 (-8.3333, 58.3333) -> (-8.3333, 75) construction
  line L504 (8.3333, 75) -> (25, 75) construction
  line L505 (25, 75) -> (25, 58.3333) construction
  line L506 (25, 58.3333) -> (8.3333, 58.3333) construction
  line L507 (8.3333, 58.3333) -> (8.3333, 75) construction
  line L508 (25, 75) -> (41.6667, 75) construction
  line L509 (41.6667, 75) -> (41.6667, 58.3333) construction
  line L510 (41.6667, 58.3333) -> (25, 58.3333) construction
  line L511 (25, 58.3333) -> (25, 75) construction
  line L512 (41.6667, 75) -> (58.3333, 75) construction
  line L513 (58.3333, 75) -> (58.3333, 58.3333) construction
  line L514 (58.3333, 58.3333) -> (41.6667, 58.3333) construction
  line L515 (41.6667, 58.3333) -> (41.6667, 75) construction
  line L516 (58.3333, 75) -> (75, 75) construction
  line L517 (75, 75) -> (75, 58.3333) construction
  line L518 (75, 58.3333) -> (58.3333, 58.3333) construction
  line L519 (58.3333, 58.3333) -> (58.3333, 75) construction
  line L520 (75, 75) -> (91.6667, 75) construction
  line L521 (91.6667, 75) -> (91.6667, 58.3333) construction
  line L522 (91.6667, 58.3333) -> (75, 58.3333) construction
  line L523 (75, 58.3333) -> (75, 75) construction
  line L524 (-91.6667, 91.6667) -> (-75, 91.6667) construction
  line L525 (-75, 91.6667) -> (-75, 75) construction
  line L526 (-75, 75) -> (-91.6667, 75) construction
  line L527 (-91.6667, 75) -> (-91.6667, 91.6667) construction
  line L528 (-75, 91.6667) -> (-58.3333, 91.6667) construction
  line L529 (-58.3333, 91.6667) -> (-58.3333, 75) construction
  line L530 (-58.3333, 75) -> (-75, 75) construction
  line L531 (-75, 75) -> (-75, 91.6667) construction
  line L532 (-58.3333, 91.6667) -> (-41.6667, 91.6667) construction
  line L533 (-41.6667, 91.6667) -> (-41.6667, 75) construction
  line L534 (-41.6667, 75) -> (-58.3333, 75) construction
  line L535 (-58.3333, 75) -> (-58.3333, 91.6667) construction
  line L536 (-41.6667, 91.6667) -> (-25, 91.6667) construction
  line L537 (-25, 91.6667) -> (-25, 75) construction
  line L538 (-25, 75) -> (-41.6667, 75) construction
  line L539 (-41.6667, 75) -> (-41.6667, 91.6667) construction
  line L540 (-25, 91.6667) -> (-8.3333, 91.6667) construction
  line L541 (-8.3333, 91.6667) -> (-8.3333, 75) construction
  line L542 (-8.3333, 75) -> (-25, 75) construction
  line L543 (-25, 75) -> (-25, 91.6667) construction
  line L544 (-8.3333, 91.6667) -> (8.3333, 91.6667) construction
  line L545 (8.3333, 91.6667) -> (8.3333, 75) construction
  line L546 (8.3333, 75) -> (-8.3333, 75) construction
  line L547 (-8.3333, 75) -> (-8.3333, 91.6667) construction
  line L548 (8.3333, 91.6667) -> (25, 91.6667) construction
  line L549 (25, 91.6667) -> (25, 75) construction
  line L550 (25, 75) -> (8.3333, 75) construction
  line L551 (8.3333, 75) -> (8.3333, 91.6667) construction
  line L552 (25, 91.6667) -> (41.6667, 91.6667) construction
  line L553 (41.6667, 91.6667) -> (41.6667, 75) construction
  line L554 (41.6667, 75) -> (25, 75) construction
  line L555 (25, 75) -> (25, 91.6667) construction
  line L556 (41.6667, 91.6667) -> (58.3333, 91.6667) construction
  line L557 (58.3333, 91.6667) -> (58.3333, 75) construction
  line L558 (58.3333, 75) -> (41.6667, 75) construction
  line L559 (41.6667, 75) -> (41.6667, 91.6667) construction
  line L560 (58.3333, 91.6667) -> (75, 91.6667) construction
  line L561 (75, 91.6667) -> (75, 75) construction
  line L562 (75, 75) -> (58.3333, 75) construction
  line L563 (58.3333, 75) -> (58.3333, 91.6667) construction
  line L564 (75, 91.6667) -> (91.6667, 91.6667) construction
  line L565 (91.6667, 91.6667) -> (91.6667, 75) construction
  line L566 (91.6667, 75) -> (75, 75) construction
  line L567 (75, 75) -> (75, 91.6667) construction
  point P0 (0, 0)
  point P1 (-83.3333, -83.3333)
  point P2 (-91.6667, -83.3333)
  point P3 (-83.3333, -75)
  point P4 (-66.6667, -83.3333)
  point P5 (-75, -83.3333)
  point P6 (-66.6667, -75)
  point P7 (-50, -83.3333)
  point P8 (-58.3333, -83.3333)
  point P9 (-50, -75)
  point P10 (-33.3333, -83.3333)
  point P11 (-41.6667, -83.3333)
  point P12 (-33.3333, -75)
  point P13 (-16.6667, -83.3333)
  point P14 (-25, -83.3333)
  point P15 (-16.6667, -75)
  point P16 (0, -83.3333)
  point P17 (-8.3333, -83.3333)
  point P18 (0, -75)
  point P19 (-83.3333, -66.6667)
  point P20 (-91.6667, -66.6667)
  point P21 (-83.3333, -58.3333)
  point P22 (-66.6667, -66.6667)
  point P23 (-75, -66.6667)
  point P24 (-66.6667, -58.3333)
  point P25 (-50, -66.6667)
  point P26 (-58.3333, -66.6667)
  point P27 (-50, -58.3333)
  point P28 (-33.3333, -66.6667)
  point P29 (-41.6667, -66.6667)
  point P30 (-33.3333, -58.3333)
  point P31 (-16.6667, -66.6667)
  point P32 (-25, -66.6667)
  point P33 (-16.6667, -58.3333)
  point P34 (0, -66.6667)
  point P35 (-8.3333, -66.6667)
  point P36 (0, -58.3333)
  point P37 (-83.3333, -50)
  point P38 (-91.6667, -50)
  point P39 (-83.3333, -41.6667)
  point P40 (-66.6667, -50)
  point P41 (-75, -50)
  point P42 (-66.6667, -41.6667)
  point P43 (-50, -50)
  point P44 (-58.3333, -50)
  point P45 (-50, -41.6667)
  point P46 (-33.3333, -50)
  point P47 (-41.6667, -50)
  point P48 (-33.3333, -41.6667)
  point P49 (-16.6667, -50)
  point P50 (-25, -50)
  point P51 (-16.6667, -41.6667)
  point P52 (0, -50)
  point P53 (-8.3333, -50)
  point P54 (0, -41.6667)
  point P55 (-83.3333, -33.3333)
  point P56 (-91.6667, -33.3333)
  point P57 (-83.3333, -25)
  point P58 (-66.6667, -33.3333)
  point P59 (-75, -33.3333)
  point P60 (-66.6667, -25)
  point P61 (-50, -33.3333)
  point P62 (-58.3333, -33.3333)
  point P63 (-50, -25)
  point P64 (-33.3333, -33.3333)
  point P65 (-41.6667, -33.3333)
  point P66 (-33.3333, -25)
  point P67 (-16.6667, -33.3333)
  point P68 (-25, -33.3333)
  point P69 (-16.6667, -25)
  point P70 (0, -33.3333)
  point P71 (-8.3333, -33.3333)
  point P72 (0, -25)
  point P73 (-83.3333, -16.6667)
  point P74 (-91.6667, -16.6667)
  point P75 (-83.3333, -8.3333)
  point P76 (-66.6667, -16.6667)
  point P77 (-75, -16.6667)
  point P78 (-66.6667, -8.3333)
  point P79 (-50, -16.6667)
  point P80 (-58.3333, -16.6667)
  point P81 (-50, -8.3333)
  point P82 (-33.3333, -16.6667)
  point P83 (-41.6667, -16.6667)
  point P84 (-33.3333, -8.3333)
  point P85 (-16.6667, -16.6667)
  point P86 (-25, -16.6667)
  point P87 (-16.6667, -8.3333)
  point P88 (0, -16.6667)
  point P89 (-8.3333, -16.6667)
  point P90 (0, -8.3333)
  point P91 (-83.3333, 0)
  point P92 (-91.6667, 0)
  point P93 (-83.3333, 8.3333)
  point P94 (-66.6667, 0)
  point P95 (-75, 0)
  point P96 (-66.6667, 8.3333)
  point P97 (-50, 0)
  point P98 (-58.3333, 0)
  point P99 (-50, 8.3333)
  point P100 (-33.3333, 0)
  point P101 (-41.6667, 0)
  point P102 (-33.3333, 8.3333)
  point P103 (-16.6667, 0)
  point P104 (-25, 0)
  point P105 (-16.6667, 8.3333)
  point P106 (0, 0)
  point P107 (-8.3333, 0)
  point P108 (0, 8.3333)
  point P109 (-83.3333, 16.6667)
  point P110 (-91.6667, 16.6667)
  point P111 (-83.3333, 25)
  point P112 (-66.6667, 16.6667)
  point P113 (-75, 16.6667)
  point P114 (-66.6667, 25)
  point P115 (-50, 16.6667)
  point P116 (-58.3333, 16.6667)
  point P117 (-50, 25)
  point P118 (-33.3333, 16.6667)
  point P119 (-41.6667, 16.6667)
  point P120 (-33.3333, 25)
  point P121 (-16.6667, 16.6667)
  point P122 (-25, 16.6667)
  point P123 (-16.6667, 25)
  point P124 (0, 16.6667)
  point P125 (-8.3333, 16.6667)
  point P126 (0, 25)
  point P127 (-83.3333, 33.3333)
  point P128 (-91.6667, 33.3333)
  point P129 (-83.3333, 41.6667)
  point P130 (-66.6667, 33.3333)
  point P131 (-75, 33.3333)
  point P132 (-66.6667, 41.6667)
  point P133 (-50, 33.3333)
  point P134 (-58.3333, 33.3333)
  point P135 (-50, 41.6667)
  point P136 (-33.3333, 33.3333)
  point P137 (-41.6667, 33.3333)
  point P138 (-33.3333, 41.6667)
  point P139 (-16.6667, 33.3333)
  point P140 (-25, 33.3333)
  point P141 (-16.6667, 41.6667)
  point P142 (0, 33.3333)
  point P143 (-8.3333, 33.3333)
  point P144 (0, 41.6667)
  point P145 (-83.3333, 50)
  point P146 (-91.6667, 50)
  point P147 (-83.3333, 58.3333)
  point P148 (-66.6667, 50)
  point P149 (-75, 50)
  point P150 (-66.6667, 58.3333)
  point P151 (-50, 50)
  point P152 (-58.3333, 50)
  point P153 (-50, 58.3333)
  point P154 (-33.3333, 50)
  point P155 (-41.6667, 50)
  point P156 (-33.3333, 58.3333)
  point P157 (-16.6667, 50)
  point P158 (-25, 50)
  point P159 (-16.6667, 58.3333)
  point P160 (0, 50)
  point P161 (-8.3333, 50)